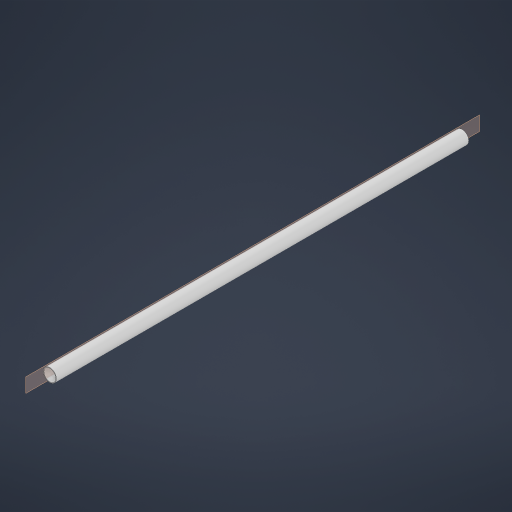
# Autodesk Inventor part: Tubo para aspersores 2
Saved by Autodesk Inventor 2024 (Build 280153000, 153)
## iProperties
Created: 2024-11-05
Part Number: Tubo para aspersores 2
Material: Genérico
Document SubType Name: Modeling
Designer: nesto
Density: 1 g/cm^3
Appearance: Valor por defecto
Author: nesto
Autodesk Inventor part; units mm, degrees
ref_plane "XZ Plane" through (0, 0, 0) normal (0, 1, 0) x (-1, 0, 0)
ref_plane "XY Plane" through (0, 0, 0) normal (0, 0, 1) x (1, 0, 0)
sketch "Boceto1" plane through (0, 0, 0) normal (0, 0, 1) x (1, 0, 0)
  circle A0 centre (0, 0) radius 95
  circle A1 centre (0, 0) radius 85.31
  dimension "d0" = 190
  dimension "d1" = 170.62
  constraints: 2 centre point, 2 coincident
  measures "d0" diameter of A0
  measures "d1" diameter of A1
extrude "Extrusión1" add sketch "Boceto1" along normal blind 6000
ref_plane "Plano de trabajo5" through (-47.5, 0, 0) normal (1, 0, 0) x (0, 1, 0)
sketch "Boceto7" plane through (-47.5, 0, 0) normal (1, 0, 0) x (0, 1, 0)
  line L0 (0, 0) -> (0, 3000) construction
  circle A0 centre (0, 3000) radius 52.5
  dimension "d22" = 105
  constraints: 2 end point, 1 centre point, 1 coincident, 1 vertical
  measures "d22" diameter of A0
extrude "Extrusión6" cut sketch "Boceto7" along normal mid plane 100
